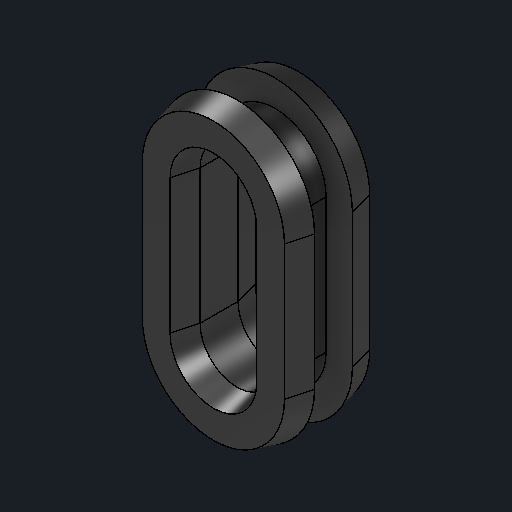
# Autodesk Inventor part: Nibblets
Saved by Autodesk Inventor 2026.2 (Build 302298000, 298)
## iProperties
Created: 2015-04-29
Part Number: Nibblets
Material: Generic
Document SubType Name: Modeling
Designer: Philip
Density: 1 g/cm^3
Appearance: Glossy - Black
Author: Philip
Autodesk Inventor part; units mm, degrees
ref_plane "YZ Plane" through (0, 0, 0) normal (1, 0, 0) x (0, 1, 0)
ref_plane "XZ Plane" through (0, 0, 0) normal (0, 1, 0) x (-1, 0, 0)
ref_plane "XY Plane" through (0, 0, 0) normal (0, 0, 1) x (1, 0, 0)
sketch "Sketch1" plane through (0, 0, 0) normal (0, 0, 1) x (1, 0, 0)
  arc A0 (2.287945, 4.093737) -> (-3.198455, 4.093737) centre (-0.455255, 4.093737) ccw
  arc A1 (-3.198455, -3.119863) -> (2.287945, -3.119863) centre (-0.455255, -3.119863) ccw
  line L0 (-3.198455, 4.093737) -> (-3.198455, -3.119863)
  line L1 (2.287945, 4.093737) -> (2.287945, -3.119863)
  arc A2 (1.525945, 4.093737) -> (-2.436455, 4.093737) centre (-0.455255, 4.093737) ccw
  line L2 (1.525945, 4.093737) -> (1.525945, -3.119863)
  arc A3 (-2.436455, -3.119863) -> (1.525945, -3.119863) centre (-0.455255, -3.119863) ccw
  line L3 (-2.436455, -3.119863) -> (-2.436455, 4.093737)
  point P0 (0, 0)
  dimension "d0" = 5.4864
  dimension "d1" = 5.4864
  dimension "d3" = 12.7
  dimension "d4" = 0.762
  constraints: 8 end point, 8 point on circle, 4 centre point, 3 tangent, 2 parallel, 1 vertical, 3 other
  measures "d0" diameter of A1
  measures "d1" diameter of A0
  measures "d4" radial gap between concentric circles of A0 A2
extrude "Extrusion1" add sketch "Sketch1" along normal mid plane 2.032
sketch "Sketch2" plane through (0, 0, 1.016) normal (0, 0, 1) x (1, 0, 0)
  line L0 (1.525945, -3.119863) -> (1.525945, 4.093737)
  arc A0 (1.525945, 4.093737) -> (-2.436455, 4.093737) centre (-0.455255, 4.093737) ccw
  line L1 (-2.436455, 4.093737) -> (-2.436455, -3.119863)
  arc A1 (-2.436455, -3.119863) -> (1.525945, -3.119863) centre (-0.455255, -3.119863) ccw
  line L2 (2.287945, 4.093737) -> (2.287945, -3.119863)
  arc A2 (-3.198455, -3.119863) -> (2.287945, -3.119863) centre (-0.455255, -3.119863) ccw
  line L3 (-3.198455, -3.119863) -> (-3.198455, 4.093737)
  arc A3 (2.287945, 4.093737) -> (-3.198455, 4.093737) centre (-0.455255, 4.093737) ccw
  arc A4 (3.697645, 4.093737) -> (-4.608155, 4.093737) centre (-0.455255, 4.093737) ccw
  line L4 (3.697645, 4.093737) -> (3.697645, -3.119863)
  arc A5 (-4.608155, -3.119863) -> (3.697645, -3.119863) centre (-0.455255, -3.119863) ccw
  line L5 (-4.608155, -3.119863) -> (-4.608155, 4.093737)
  point P0 (0, 0)
  dimension "d7" = 8.3058
  constraints: 4 end point, 4 point on circle, 2 centre point, 3 other
  measures "d7" distance between parallel lines of L4 L5
sketch "Sketch2 outline for Extrusion2" plane through (0, 0, 1.016) normal (0, 0, 1) x (1, 0, 0)
  arc A0 (-4.608155, 4.093737) -> (3.697645, 4.093737) centre (-0.455255, 4.093737) cw
  line L0 (-4.608155, -3.119863) -> (-4.608155, 4.093737)
  line L1 (3.697645, 4.093737) -> (3.697645, -3.119863)
  arc A1 (3.697645, -3.119863) -> (-4.608155, -3.119863) centre (-0.455255, -3.119863) cw
  arc A2 (-2.436455, -3.119863) -> (1.525945, -3.119863) centre (-0.455255, -3.119863) ccw
  line L2 (1.525945, -3.119863) -> (1.525945, 4.093737)
  arc A3 (1.525945, 4.093737) -> (-2.436455, 4.093737) centre (-0.455255, 4.093737) ccw
  line L3 (-2.436455, 4.093737) -> (-2.436455, -3.119863)
extrude "Extrusion2" add sketch "Sketch2 outline for Extrusion2" along normal blind 1.27 draft -15
mirror "Mirror1" about plane through (0, 0, 0) normal (0, 0, 1) of "Extrusion2"
body "Solid1"
